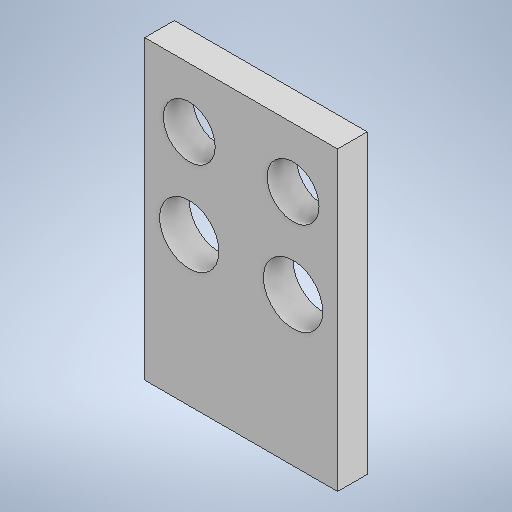
# Autodesk Inventor part: N20shaft_sizing
Saved by Autodesk Inventor 2025.2 (Build 292293000, 293)
## iProperties
Created: 2025-03-05
Part Number: N20shaft_sizing
Material: Generic
Document SubType Name: Modeling
Designer: 3lin2
Density: 1 g/cm^3
Appearance: Default
Author: 3lin2
Autodesk Inventor part; units mm, degrees
ref_plane "YZ Plane" through (0, 0, 0) normal (1, 0, 0) x (0, 1, 0)
ref_plane "XZ Plane" through (0, 0, 0) normal (0, 1, 0) x (-1, 0, 0)
ref_plane "XY Plane" through (0, 0, 0) normal (0, 0, 1) x (1, 0, 0)
sketch "Sketch1" plane through (0, 0, 0) normal (0, 0, 1) x (1, 0, 0)
  line L0 (-9.9986, 9.999) -> (3.0014, 9.999)
  line L1 (3.0014, 9.999) -> (3.0014, -10.001)
  line L2 (3.0014, -10.001) -> (-9.9986, -10.001)
  line L3 (-9.9986, -10.001) -> (-9.9986, 9.999)
  point P0 (0.0014, -0.001)
  point P1 (0.0014, -0.001)
  point P2 (-9.9986, -0.001)
  dimension "d0" = 13
  dimension "d1" = 20
  dimension "d2" = 10
  dimension "d3" = 10
  constraints: 8 end point, 2 parallel, 1 coincident, 1 horizontal, 1 midpoint, 1 perpendicular
  measures "d0" distance between parallel lines of L1 L3
  measures "d1" distance between parallel lines of L2 L0
  measures "d2" distance of point (-9.999, -0.001) point (0.001, -0.001)
  measures "d3" distance from line of point (0.001, -0.001) L0
extrude "Extrusion1" add sketch "Sketch1" along normal blind 2
sketch "Sketch4" plane through (0, 0, 2) normal (0, 0, 1) x (1, 0, 0)
  line L0 (3.0014, 9.999) -> (-9.9986, 9.999) projected
  line L1 (-9.9986, 9.999) -> (-9.9986, -10.001) projected
  point P0 (-6.9986, 5.999)
  point P1 (0.0014, 5.999)
  dimension "d20" = 4
  dimension "d21" = 3
  dimension "d29" = 4
  measures "d20" distance from line of point (-6.999, 5.999) L0
  measures "d21" distance from line of L1 point (-6.999, 5.999)
  measures "d29" distance from line of L0 point (0.001, 5.999)
hole "Hole3" at (-6.9986, 5.999, 2) at (0.0014, 5.999, 2) direction (0, 0, -1) diameter 3.5 end through all
sketch "Sketch5" plane through (0, 0, 2) normal (0, 0, 1) x (1, 0, 0)
  line L0 (-9.9986, 9.999) -> (-9.9986, -10.001) projected
  point P0 (0, 0)
  point P1 (-6.9986, 0)
  point P2 (0, 0)
  point P3 (-9.9986, -0.001)
  dimension "d37" = 3
  constraints: 1 coincident, 1 midpoint
  measures "d37" distance of point (-9.999, -0.001) point (-6.999, 0)
hole "Hole4" at (-6.9986, 0, 2) at (0, 0, 2) direction (0, 0, -1) diameter 4 end through all
body "Solid1"
